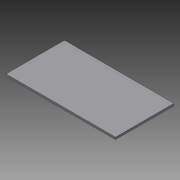
# Autodesk Inventor part: Frount
Saved by Autodesk Inventor 2015 (Build 190159000, 159)
## iProperties
Created: 2014-11-13
Part Number: Frount
Material: Generic
Document SubType Name: Modeling
Designer: karl
Density: 1 g/cm^3
Appearance: Default
Author: karl
Autodesk Inventor part; units mm, degrees
ref_plane "YZ Plane" through (0, 0, 0) normal (1, 0, 0) x (0, 1, 0)
ref_plane "XZ Plane" through (0, 0, 0) normal (0, 1, 0) x (-1, 0, 0)
ref_plane "XY Plane" through (0, 0, 0) normal (0, 0, 1) x (1, 0, 0)
sketch "Sketch1" plane through (0, 0, 0) normal (0, 0, 1) x (1, 0, 0)
  line L0 (-91.239, 32) -> (-91.239, 35) projected
  line L1 (51.239, 32) -> (51.239, 35) projected
  line L2 (51.239, -41) -> (51.239, -38) projected
  line L3 (-91.239, 35) -> (51.239, 35)
  line L4 (51.239, 35) -> (51.239, -41)
  line L5 (51.239, -41) -> (-91.239, -41)
  line L6 (-91.239, -41) -> (-91.239, 35)
  point P0 (0, 0)
  constraints: 8 end point, 2 parallel, 1 horizontal, 1 perpendicular
extrude "Extrusion1" add sketch "Sketch1" against normal blind 3
sketch "Sketch2" plane through (0, 0, 0) normal (0, 0, 1) x (1, 0, 0)
  line L0 (-80, 35) -> (-80, 32) projected
  line L1 (-80, 32) -> (-50, 32) projected
  line L2 (-50, 32) -> (-50, 35) projected
  line L3 (-80, 35) -> (-50, 35) projected
  line L4 (-10, 32) -> (-10, 35) projected
  line L5 (-30, 35) -> (-10, 35) projected
  line L6 (-30, 35) -> (-30, 32) projected
  line L7 (-30, 32) -> (-10, 32) projected
  line L8 (-50, 0) -> (-70, 0) projected
  line L9 (-70, 0) -> (-70, -3) projected
  line L10 (-70, -3) -> (-50, -3) projected
  line L11 (-50, 0) -> (-50, -3) projected
  line L12 (-30, 0) -> (-40, 0) projected
  line L13 (-40, 0) -> (-40, -3) projected
  line L14 (-40, -3) -> (-30, -3) projected
  line L15 (-30, 0) -> (-30, -3) projected
  line L16 (-80, -28) -> (-80, -18) projected
  line L17 (-80, -28) -> (-77, -28) projected
  line L18 (-77, -18) -> (-77, -28) projected
  line L19 (-80, -18) -> (-77, -18) projected
  line L20 (-80, 2) -> (-80, 22) projected
  line L21 (-80, 2) -> (-77, 2) projected
  line L22 (-77, 22) -> (-77, 2) projected
  line L23 (-80, 22) -> (-77, 22) projected
  line L24 (-80, -41) -> (-80, -38) projected
  line L25 (-91.239, -38) -> (-80, -38) projected
  line L26 (-91.239, -41) -> (-91.239, -38) projected
  line L27 (-91.239, -41) -> (-80, -41) projected
  line L28 (-40, -41) -> (-40, -38) projected
  line L29 (-60, -38) -> (-40, -38) projected
  line L30 (-60, -38) -> (-60, -41) projected
  line L31 (-60, -41) -> (-40, -41) projected
  line L32 (-10, -41) -> (-10, -38) projected
  line L33 (-30, -38) -> (-10, -38) projected
  line L34 (-30, -38) -> (-30, -41) projected
  line L35 (-30, -41) -> (-10, -41) projected
  point P0 (0, 0)
extrude "Extrusion2" cut sketch "Sketch2" against normal blind 3 contours L3 L2 L1 L0 | L7 L6 L5 L4 | L11 L10 L9 L8 | L15 L14 L13 L12 | L20 L23 L22 L21 | L27 L26 L25 L24 | L31 L30 L29 L28 | L35 L34 L33 L32
sketch "Sketch3" plane through (0, 0, 0) normal (0, 0, 1) x (1, 0, 0)
  line L0 (-90, 32) -> (-90, 35) projected
  line L1 (-91.239, 35) -> (-90, 35) projected
  line L2 (-91.239, 32) -> (-91.239, 35) projected
  line L3 (-91.239, 32) -> (-90, 32) projected
  line L4 (-87.5, -3) -> (-82.5, -3) projected
  line L5 (-87.5, -6) -> (-82.5, -6) projected
  line L6 (-82.5, -6) -> (-82.5, -3) projected
  line L7 (-87.5, -6) -> (-87.5, -3) projected
  line L8 (-77, -18) -> (-77, -28) projected
  line L9 (-80, -28) -> (-80, -18) projected
  line L10 (-80, -18) -> (-77, -18) projected
  line L11 (-80, -28) -> (-77, -28) projected
  line L12 (-55, -10.5) -> (-55, -30.5) projected
  line L13 (-55, -10.5) -> (-58, -10.5) projected
  line L14 (-58, -30.5) -> (-58, -10.5) projected
  line L15 (-55, -30.5) -> (-58, -30.5) projected
  point P0 (0, 0)
extrude "Extrusion3" cut sketch "Sketch3" against normal blind 3
ref_plane "Work Plane1" through (-20, -41, 0) normal (1, 0, 0) x (0, 0, -1)
mirror "Mirror1" about plane through (-20, -41, 0) normal (1, 0, 0) of "Extrusion3", "Extrusion2"
body "Solid1"
